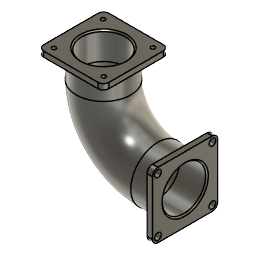
Flanged Elbow (Autodesk Fusion 360 design; units mm, degrees)
part number: 2026-01-02-03-20-00-913
Autodesk Fusion 360 part; units mm, degrees
sketch "Sketch1" plane through (0, 0, 0) normal (0, 1, 0) x (1, 0, 0)
  line L0 (0, -100) -> (0, -150)
  line L1 (100, 0) -> (150, 0)
  arc A0 (100, 0) -> (0, -100) centre (100, -100) ccw
  dimension "d1" = 150
  dimension "d2" = 150
  dimension "d3" = 100
  constraint perpendicular L0 L1
  constraint coincident origin L0
  constraint coincident origin L1
  constraint tangent L0 A0
  constraint tangent L1 A0
  measures "d1" distance of origin L0.end
  measures "d2" distance of origin L1.end
  measures "d3" radius of A0
pipe "Pipe1" add diameter 100 wall 10 path "Sketch1" along L0 A0 L1
sketch "Sketch2" plane through (150, 0, 0) normal (1, 0, 0) x (0, 1, 0)
  circle A0 centre (0, 0) radius 40
  circle A1 centre (0, 0) radius 50
  line L0 (50, 60) -> (-50, 60)
  line L1 (-60, 50) -> (-60, -50)
  line L2 (-50, -60) -> (50, -60)
  line L3 (60, -50) -> (60, 50)
  line L4 (60, 60) -> (-60, -60) construction
  line L5 (-60, 60) -> (60, -60) construction
  arc A2 (60, 50) -> (50, 60) centre (50, 50) ccw
  arc A3 (-50, 60) -> (-60, 50) centre (-50, 50) ccw
  arc A4 (-60, -50) -> (-50, -60) centre (-50, -50) ccw
  arc A5 (50, -60) -> (60, -50) centre (50, -50) ccw
  circle A6 centre (50, -50) radius 6.25
  circle A7 centre (50, 50) radius 6.25
  circle A8 centre (-50, 50) radius 6.25
  circle A9 centre (-50, -50) radius 6.25
  dimension "d8" = 120
  dimension "d9" = 120
  dimension "d10" = 10
  dimension "d11" = 10
  dimension "d12" = 10
  dimension "d13" = 12.5
  dimension "d18" = 10
  dimension "d20" = 360
  constraint horizontal L0
  constraint perpendicular L0 L1
  constraint parallel L0 L2
  constraint parallel L1 L3
  constraint coincident L4 A0.centre
  constraint coincident L5 A0.centre
  constraint coincident A0.centre A1.centre
  constraint coincident L4.start L3
  constraint coincident L4.start L0
  constraint tangent L3 A2
  constraint tangent L0 A2
  constraint coincident L5.start L0
  constraint coincident L5.start L1
  constraint tangent L0 A3
  constraint tangent L1 A3
  constraint coincident L4.end L1
  constraint coincident L4.end L2
  constraint tangent L1 A4
  constraint tangent L2 A4
  constraint equal A3 A4
  constraint coincident L5.end L3
  constraint coincident L5.end L2
  constraint tangent L3 A5
  constraint tangent L2 A5
  constraint concentric A5 A6
  measures "d8" distance of L4.end L5.end
  measures "d9" distance of L5.start L4.end
  measures "d10" radius of A2
  measures "d11" radius of A3
  measures "d12" radius of A5
  measures "d13" diameter of A6
  measures "d18" distance of L3 A5.centre
sketch "Sketch3" plane through (0, 0, 0) normal (1, 0, 0) x (0, 1, 0)
  circle A0 centre (50, -50) radius 6.25
  line L0 (60, -50) -> (60, 50)
  point P0 (50, -50)
  dimension "d15" = 12.5
  dimension "d16" = 10
  measures "d15" diameter of A0
  measures "d16" distance of P0 L0
sketch "Sketch4" plane through (0, 0, 0) normal (1, 0, 0) x (0, 1, 0)
  line L0 (60, -50) -> (60, 50)
  point P0 (50, -50)
  dimension "d17" = 10
  measures "d17" distance of P0 L0
sketch "Sketch5" plane through (150, 0, 0) normal (1, 0, 0) x (0, 1, 0)
extrude "Extrude1" add sketch "Sketch2" against normal blind 10 contours L0 L1 L2 L3 A2 A3 A4 A5
sketch "Sketch6" plane through (0, 0, 150) normal (0, 0, 1) x (-1, 0, 0)
  circle A0 centre (0, 0) radius 40
  circle A1 centre (0, 0) radius 50
  line L0 (50, 60) -> (-50, 60)
  line L1 (-60, 50) -> (-60, -50)
  line L2 (-50, -60) -> (50, -60)
  line L3 (60, -50) -> (60, 50)
  line L4 (60, 60) -> (-60, -60) construction
  line L5 (-60, 60) -> (60, -60) construction
  arc A2 (60, 50) -> (50, 60) centre (50, 50) ccw
  arc A3 (-50, 60) -> (-60, 50) centre (-50, 50) ccw
  arc A4 (-60, -50) -> (-50, -60) centre (-50, -50) ccw
  arc A5 (50, -60) -> (60, -50) centre (50, -50) ccw
  circle A6 centre (-45, 45) radius 6.25
  circle A7 centre (-45, -45) radius 6.25
  circle A8 centre (45, -45) radius 6.25
  circle A9 centre (45, 45) radius 6.25
  dimension "d23" = 120
  dimension "d24" = 120
  dimension "d25" = 10
  dimension "d26" = 12.5
  dimension "d27" = 15
  dimension "d29" = 360
  constraint horizontal L0
  constraint perpendicular L0 L1
  constraint parallel L0 L2
  constraint parallel L1 L3
  constraint coincident L4 A0.centre
  constraint coincident L5 A0.centre
  constraint coincident A0.centre A1.centre
  constraint coincident L4.start L0
  constraint coincident L4.start L3
  constraint tangent L0 A2
  constraint tangent L3 A2
  constraint coincident L5.start L1
  constraint coincident L5.start L0
  constraint tangent L1 A3
  constraint tangent L0 A3
  constraint equal A2 A3
  constraint coincident L4.end L1
  constraint coincident L4.end L2
  constraint tangent L1 A4
  constraint tangent L2 A4
  constraint equal A2 A4
  constraint coincident L5.end L2
  constraint coincident L5.end L3
  constraint tangent L2 A5
  constraint tangent L3 A5
  constraint equal A2 A5
  constraint coincident L5 A6.centre
  measures "d23" distance of L4.end L5.end
  measures "d24" distance of L5.start L4.end
  measures "d25" radius of A2
  measures "d26" diameter of A6
  measures "d27" distance of L1 A6.centre
extrude "Extrude2" add sketch "Sketch6" against normal blind 10 contours L0 L1 L2 L3 A2 A3 A4 A5 | A6 | A7 | A8 | A9
hole "Hole1" at (-45.7626, 45.1236, 150) direction (0, 0, -1) diameter 7.5 depth 10 tip angle 180
pattern_circular "C-Pattern1" count 4 over 360 about axis through (0, 0, 150) along (0, 0, 1) of "Hole1"
chamfer "Chamfer1" distance 2.5 angle 45 2 edges at (37.2931, -14.4646, 150) (150, 14.4646, 37.2931)
